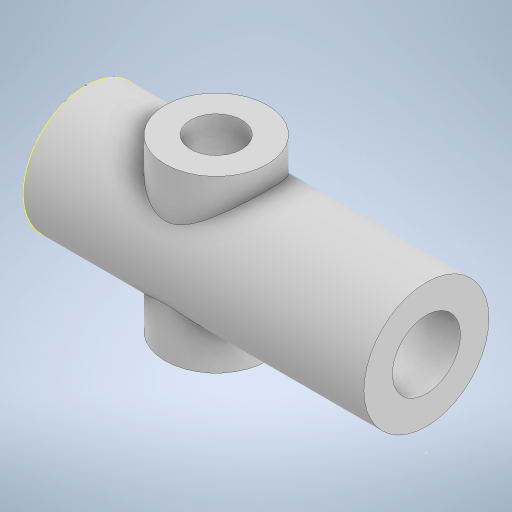
# Autodesk Inventor part: codo
Saved by Autodesk Inventor 2024 (Build 280153000, 153)
## iProperties
Created: 2024-03-24
Part Number: codo
Material: Generic
Document SubType Name: Modeling
Designer: JDAM
Density: 1 g/cm^3
Appearance: Default
Author: JDAM
Autodesk Inventor part; units mm, degrees
ref_plane "XZ Plane" through (0, 0, 0) normal (0, 1, 0) x (-1, 0, 0)
ref_plane "XY Plane" through (0, 0, 0) normal (0, 0, 1) x (1, 0, 0)
sketch "Sketch1" plane through (0, 0, 0) normal (0, 1, 0) x (-1, 0, 0)
  circle A0 centre (0, 0) radius 2.2
  circle A1 centre (0, 0) radius 4.5
  dimension "d0" = 4.4
  dimension "d1" = 9
  constraints: 2 centre point, 2 coincident
  measures "d0" diameter of A0
  measures "d1" diameter of A1
extrude "Extrusion1" add sketch "Sketch1" along normal blind 15 contours A0 | A1
sketch "Sketch2" plane through (0, 15, 0) normal (0, 1, 0) x (1, 0, 0)
  circle A0 centre (0, 0) radius 2.2
  dimension "d4" = 4.4
  constraints: 1 centre point, 1 coincident
  measures "d4" diameter of A0
ref_plane "Work Plane1" through (3.5, 0, 0) normal (1, 0, 0) x (0, 1, 0)
sketch "Sketch3" plane through (3.5, 0, 0) normal (1, 0, 0) x (0, 1, 0)
  line L0 (0, 0) -> (7.5, 0)
  circle A0 centre (7.5, 0) radius 5.5
  dimension "d13" = 7.5
  dimension "d15" = 11
  constraints: 2 end point, 1 centre point, 1 horizontal
  measures "d13" distance of L0.start L0.end
  measures "d15" diameter of A0
extrude "Extrusion2" add sketch "Sketch3" along normal mid plane 30
sketch "Sketch6" plane through (-11.5, 0, 0) normal (-1, 0, 0) x (0, 0, 1)
  circle A0 centre (0, 7.5) radius 5.5 projected
  arc A1 (0, 11) -> (0, 4) centre (0, 7.5) ccw
  line L0 (0, 2) -> (0, 13) projected
  line L1 (0, 11) -> (0, 4)
  point P0 (0, 0)
  constraints: 2 end point, 2 point on circle, 1 centre point, 1 collinear
sketch "Sketch7" plane through (18.5, 7.5, 0) normal (1, 0, 0) x (0, 0, -1)
  point P0 (0, -7.5)
hole "Hole4" at (0, 15, 0) direction (0, -1, 0) diameter 4.5 depth 20
sketch "Sketch8" plane through (18.5, 7.5, 0) normal (1, 0, 0) x (0, 0, -1)
  circle A0 centre (0, 0) radius 3
  point P0 (0, -7.5)
  dimension "d44" = 6
  constraints: 1 centre point
  measures "d44" diameter of A0
hole "Hole5" at (18.5, 7.5, 0) direction (-1, 0, 0) diameter 6 depth 15
body "Solid1"
